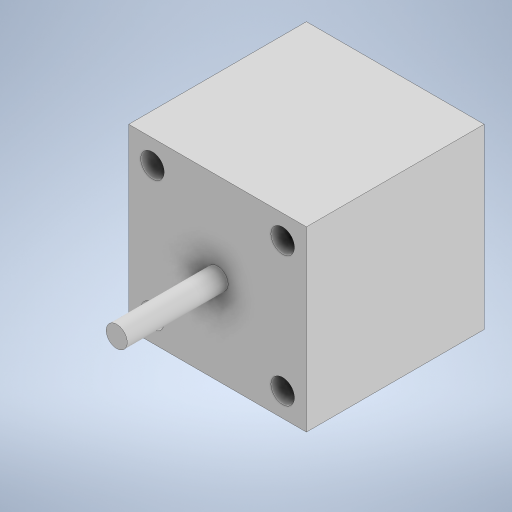
# Autodesk Inventor part: Nema 17
Saved by Autodesk Inventor 2024 (Build 280153000, 153)
## iProperties
Created: 2024-01-25
Part Number: Nema 17
Material: Generic
Document SubType Name: Modeling
Designer: aidan
Density: 1 g/cm^3
Appearance: Default
Author: aidan
Autodesk Inventor part; units mm, degrees
ref_plane "YZ Plane" through (0, 0, 0) normal (1, 0, 0) x (0, 1, 0)
ref_plane "XZ Plane" through (0, 0, 0) normal (0, 1, 0) x (-1, 0, 0)
ref_plane "XY Plane" through (0, 0, 0) normal (0, 0, 1) x (1, 0, 0)
sketch "Sketch1" plane through (0, 0, 0) normal (0, 0, 1) x (1, 0, 0)
  line L0 (0, 0) -> (-42.291, 0)
  line L1 (-42.291, 0) -> (-42.291, 42.291)
  line L2 (-42.291, 42.291) -> (0, 42.291)
  line L3 (0, 42.291) -> (0, 0)
  dimension "d0" = 42.291
  dimension "d1" = 42.291
  constraints: 8 end point, 2 parallel, 1 horizontal, 1 perpendicular
  measures "d0" distance of L2.end L0.start
  measures "d1" distance of L0.start L0.end
extrude "Extrusion1" add sketch "Sketch1" along normal blind 42.291
sketch "Sketch2" plane through (0, 0, 42.291) normal (0, 0, 1) x (1, 0, 0)
  line L0 (0, 42.291) -> (-42.291, 42.291) projected
  line L1 (-42.291, 42.291) -> (-42.291, 0) projected
  line L2 (-42.291, 0) -> (0, 0) projected
  line L3 (0, 0) -> (0, 42.291) projected
  line L4 (-5.6515, 5.6515) -> (-36.6395, 5.6515)
  line L5 (-36.6395, 5.6515) -> (-36.6395, 36.6395)
  line L6 (-36.6395, 36.6395) -> (-5.6515, 36.6395)
  line L7 (-5.6515, 36.6395) -> (-5.6515, 5.6515)
  line L8 (-5.6515, 5.6515) -> (-36.6395, 36.6395) construction
  line L9 (-36.6395, 5.6515) -> (-5.6515, 36.6395) construction
  circle A0 centre (-5.6515, 5.6515) radius 2.794
  circle A1 centre (-36.6395, 5.6515) radius 2.794
  circle A2 centre (-36.6395, 36.6395) radius 2.794
  circle A3 centre (-5.6515, 36.6395) radius 2.794
  point P0 (-21.1455, 21.1455)
  dimension "d4" = 30.988
  dimension "d5" = 30.988
  dimension "d8" = 5.588
  dimension "d9" = 5.588
  dimension "d10" = 5.588
  dimension "d11" = 5.588
  constraints: 12 end point, 4 centre point, 3 coincident, 2 midpoint, 2 parallel, 1 horizontal, 1 perpendicular
  measures "d4" distance of L5.end L6.end
  measures "d5" distance of L6.end L4.start
  measures "d8" diameter of A0
  measures "d9" diameter of A1
  measures "d10" diameter of A2
  measures "d11" diameter of A3
extrude "Extrusion2" cut sketch "Sketch2" against normal blind 68.834 contours A1 L5 L4 | L4 L5 A1 | A0 L7 L4 | L4 L7 A0 | A2 L6 L5 | L5 L6 A2 | A3 L6 L7 | L7 L6 A3
sketch "Sketch3" plane through (0, 0, 42.291) normal (0, 0, 1) x (1, 0, 0)
  circle A0 centre (-5.6515, 5.6515) radius 2.794 projected
  circle A1 centre (-5.6515, 36.6395) radius 2.794 projected
  circle A2 centre (-36.6395, 5.6515) radius 2.794 projected
  circle A3 centre (-36.6395, 36.6395) radius 2.794 projected
  line L0 (0, 42.291) -> (-42.291, 42.291) projected
  line L1 (-42.291, 42.291) -> (-42.291, 0) projected
  line L2 (-42.291, 0) -> (0, 0) projected
  line L3 (0, 0) -> (0, 42.291) projected
  circle A4 centre (-21.1455, 21.1455) radius 2.5019
  dimension "d14" = 5.0038
  constraints: 1 centre point
  measures "d14" diameter of A4
extrude "Extrusion3" add sketch "Sketch3" along normal blind 24.003 contours A4
body "Solid1"
